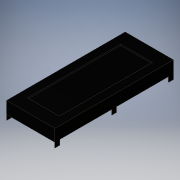
# Autodesk Inventor part: LCD_Screen
Saved by Autodesk Inventor 2016 (Build 200138000, 138)
## iProperties
Created: 2016-04-06
Part Number: LCD_Screen
Material: Steel, Mild
Document SubType Name: Modeling
Designer: agmle
Mass: 297.765 g
Surface Area: 103.657 cm^2
Volume: 37.9319 cm^3
Density: 7.85 g/cm^3
Appearance: Anodized - Black
LCD_Screen_Height: 1.555 in
LCD_Screen_Width: 3.819 in
LCD_Screen_Depth: 0.390 in
LCD_Viewable_Height: 1.024 in
LCD_Viewable_Width: 2.992 in
LCD_Screen_Tab_Width: 0.010 in
LCD_Screen_Tab_Length: 0.157 in
LCD_Screen_Tab_Depth: 0.161 in
Author: agmle
Autodesk Inventor part; units mm, degrees
ref_plane "YZ Plane" through (0, 0, 0) normal (1, 0, 0) x (0, 1, 0)
ref_plane "XZ Plane" through (0, 0, 0) normal (0, 1, 0) x (-1, 0, 0)
ref_plane "XY Plane" through (0, 0, 0) normal (0, 0, 1) x (1, 0, 0)
sketch "Sketch1" plane through (0, 0, 0) normal (0, 1, 0) x (-1, 0, 0)
  line L0 (39.5135, 44.2255) -> (0.0135, 44.2255)
  line L1 (0.0135, 44.2255) -> (0.0135, -52.7745)
  line L2 (0.0135, -52.7745) -> (39.5135, -52.7745)
  line L3 (39.5135, -52.7745) -> (39.5135, 44.2255)
  point P0 (0, 0)
  dimension "LCD_Screen_Width" = 97
  dimension "LCD_Screen_Height" = 39.5
  constraints: 8 end point, 2 parallel, 1 horizontal, 1 perpendicular
  measures "LCD_Screen_Width" distance of L2.end L0.start
  measures "LCD_Screen_Height" distance of L0.start L0.end
extrude "Extrusion1" add sketch "Sketch1" along normal blind 9.9
sketch "Sketch2" plane through (0, 9.9, 0) normal (0, 1, 0) x (1, 0, 0)
  line L0 (-32.7635, -33.7255) -> (-6.7635, -33.7255)
  line L1 (-6.7635, -33.7255) -> (-6.7635, 42.2745)
  line L2 (-6.7635, 42.2745) -> (-32.7635, 42.2745)
  line L3 (-32.7635, 42.2745) -> (-32.7635, -33.7255)
  line L4 (-39.5135, 52.7745) -> (-39.5135, -44.2255) construction
  line L5 (-39.5135, 4.2745) -> (-32.7635, 4.2745) construction
  line L6 (-6.7635, 4.2745) -> (-0.0135, 4.2745) construction
  line L7 (-0.0135, -44.2255) -> (-0.0135, 52.7745) construction
  point P0 (0, 0)
  dimension "LCD_Viewable_Height" = 26
  dimension "LCD_Viewable_Width" = 76
  constraints: 12 end point, 4 midpoint, 2 collinear, 2 parallel, 1 horizontal, 1 perpendicular
  measures "LCD_Viewable_Height" distance of L0.start L0.end
  measures "LCD_Viewable_Width" distance of L0.end L1.end
extrude "Extrusion2" cut sketch "Sketch2" against normal blind 1
sketch "Sketch3" plane through (0, 0, 0) normal (0, -1, 0) x (1, 0, 0)
  line L0 (-0.0135, 44.2255) -> (-0.2635, 44.2255)
  line L1 (-0.2635, 44.2255) -> (-0.2635, 40.2255)
  line L2 (-0.2635, 40.2255) -> (-0.0135, 40.2255)
  line L3 (-0.0135, 40.2255) -> (-0.0135, 44.2255)
  line L4 (-0.0135, -2.2745) -> (-0.2635, -2.2745)
  line L5 (-0.2635, -2.2745) -> (-0.2635, -6.2745)
  line L6 (-0.2635, -6.2745) -> (-0.0135, -6.2745)
  line L7 (-0.0135, -6.2745) -> (-0.0135, -2.2745)
  line L8 (-0.0135, -48.7745) -> (-0.2635, -48.7745)
  line L9 (-0.2635, -48.7745) -> (-0.2635, -52.7745)
  line L10 (-0.2635, -52.7745) -> (-0.0135, -52.7745)
  line L11 (-0.0135, -52.7745) -> (-0.0135, -48.7745)
  line L12 (-39.2635, -48.7745) -> (-39.5135, -48.7745)
  line L13 (-39.5135, -48.7745) -> (-39.5135, -52.7745)
  line L14 (-39.5135, -52.7745) -> (-39.2635, -52.7745)
  line L15 (-39.2635, -52.7745) -> (-39.2635, -48.7745)
  line L16 (-39.2635, -2.2745) -> (-39.5135, -2.2745)
  line L17 (-39.5135, -2.2745) -> (-39.5135, -6.2745)
  line L18 (-39.5135, -6.2745) -> (-39.2635, -6.2745)
  line L19 (-39.2635, -6.2745) -> (-39.2635, -2.2745)
  line L20 (-39.2635, 44.2255) -> (-39.5135, 44.2255)
  line L21 (-39.5135, 44.2255) -> (-39.5135, 40.2255)
  line L22 (-39.5135, 40.2255) -> (-39.2635, 40.2255)
  line L23 (-39.2635, 40.2255) -> (-39.2635, 44.2255)
  line L24 (-0.0135, 44.2255) -> (-0.0135, -52.7745) projected
  line L25 (-39.5135, -52.7745) -> (-39.5135, 44.2255) projected
  line L26 (-39.5135, 44.2255) -> (-0.0135, 44.2255) projected
  line L27 (-0.0135, -52.7745) -> (-39.5135, -52.7745) projected
  line L28 (-0.2635, 40.2255) -> (-0.2635, -2.2745) construction
  line L29 (-0.2635, -6.2745) -> (-0.2635, -48.7745) construction
  point P0 (0, 0)
  dimension "LCD_Screen_Tab_Width" = 0.25
  dimension "LCD_Screen_Tab_Length" = 4
  constraints: 52 end point, 22 equal length, 8 collinear, 6 horizontal, 6 perpendicular, 5 point on line, 1 vertical
  measures "LCD_Screen_Tab_Width" distance of L0.start L0.end
  measures "LCD_Screen_Tab_Length" distance of L0.end L1.end
extrude "Extrusion3" add sketch "Sketch3" along normal blind 4.1 contours L3 L2 L1 L0 | L23 L22 L21 L20 | L7 L6 L5 L4 | L11 L10 L9 L8 | L16 L19 L18 L17 | L12 L15 L14 L13
body "Solid1"
